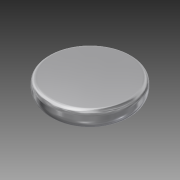
# Autodesk Inventor part: SuperCap_PAS614L
Saved by Autodesk Inventor 2014 (Build 180170000, 170)
## iProperties
Created: 2014-11-22
Part Number: SuperCap_PAS614L
Material: Silver
Document SubType Name: Modeling
Designer: DV
Mass: 0.588391 g
Surface Area: 0.995266 cm^2
Volume: 0.0560906 cm^3
Density: 10.49 g/cm^3
Appearance: Silver
Author: DV
Autodesk Inventor part; units mm, degrees
ref_plane "YZ Plane" through (0, 0, 0) normal (1, 0, 0) x (0, 1, 0)
ref_plane "XZ Plane" through (0, 0, 0) normal (0, 1, 0) x (-1, 0, 0)
ref_plane "XY Plane" through (0, 0, 0) normal (0, 0, 1) x (1, 0, 0)
sketch "Sketch1" plane through (0, 0, 0) normal (0, 0, 1) x (1, 0, 0)
  line L0 (0, 0) -> (3.019, 0)
  line L1 (3.4, -0.381) -> (3.4, -0.6409)
  line L2 (0, -1.8) -> (0, 0)
  line L3 (0, -1.8) -> (2.2393, -1.8)
  line L4 (2.3663, -1.673) -> (2.3663, -1.4282)
  line L5 (0, -1.3716) -> (0, -1.8)
  arc A0 (3.4, -0.381) -> (3.019, 0) centre (3.019, -0.381) ccw
  line L6 (2.4387, -1.5299) -> (2.511, -1.5299)
  arc A1 (2.511, -1.5299) -> (3.4, -0.6409) centre (2.511, -0.6409) ccw
  arc A2 (2.2393, -1.8) -> (2.3663, -1.673) centre (2.2393, -1.673) ccw
  line L7 (2.4387, -1.5299) -> (2.4387, -1.4282)
  line L8 (2.4387, -1.4282) -> (2.3663, -1.4282)
  point P0 (3.4, 0)
  dimension "d2" = 0.381
  dimension "d3" = 0.889
  dimension "d4" = 0.127
  constraints: 18 end point, 6 point on circle, 6 tangent, 3 centre point, 3 perpendicular, 2 horizontal, 2 parallel, 2 point on line
  measures "d2" radius of A0
  measures "d3" radius of A1
  measures "d4" radius of A2
revolve "Revolution1" add sketch "Sketch1" angle 360 about axis through (0, -1.8, 0) along (0, 1, 0)
body "Solid1"
